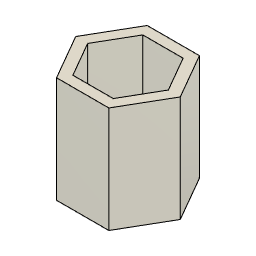
GoBilda8mmRexBoreToRev5mmHexAxleAdapter (Autodesk Fusion 360 design; units mm, degrees)
Autodesk Fusion 360 part; units mm, degrees
sketch "Sketch1" plane through (0, 0, 0) normal (0, 1, 0) x (1, 0, 0)
  line L0 (1.5588, -2.7) -> (3.1177, 0)
  line L1 (3.1177, 0) -> (1.5588, 2.7)
  line L2 (1.5588, 2.7) -> (-1.5588, 2.7)
  line L3 (-1.5588, 2.7) -> (-3.1177, 0)
  line L4 (-3.1177, 0) -> (-1.5588, -2.7)
  line L5 (-1.5588, -2.7) -> (1.5588, -2.7)
  line L6 (-4.0415, 0) -> (-2.0207, -3.5)
  line L7 (-2.0207, -3.5) -> (2.0207, -3.5)
  line L8 (2.0207, -3.5) -> (4.0415, 0)
  line L9 (4.0415, 0) -> (2.0207, 3.5)
  line L10 (2.0207, 3.5) -> (-2.0207, 3.5)
  line L11 (-2.0207, 3.5) -> (-4.0415, 0)
  dimension "d2" = 5.4
  dimension "d3" = 0.8
  dimension "d6" = 7
  dimension "d8" = 6.2354
  measures "d2" distance of L2 L5
  measures "d6" distance of L7 L10
  measures "d8" distance of L0.start L2.end
extrude "Extrude1" add sketch "Sketch1" along normal blind 8.2
